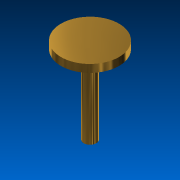
# Autodesk Inventor part: Omron SS-01GL2-E Microswitch Roller Pin
Saved by Autodesk Inventor 2016 (Build 200138000, 138)
## iProperties
Created: 2012-05-23
Material: Brass
Document SubType Name: Modeling
Designer: sdarley
Density: 1 g/cm^3
Project: Microswitch - Omron SS-01GL2-E
Description: Omron SS-01GL2-E Microswitch Roller Pin
Appearance: Brass - Polished
Author: sdarley
Title: Omron SS-01GL2-E Microswitch Roller Pin
Revision Number: 1
Autodesk Inventor part; units mm, degrees
ref_plane "YZ Plane" through (0, 0, 0) normal (1, 0, 0) x (0, 1, 0)
ref_plane "XZ Plane" through (0, 0, 0) normal (0, 1, 0) x (-1, 0, 0)
ref_plane "XY Plane" through (0, 0, 0) normal (0, 0, 1) x (1, 0, 0)
sketch "Sketch1" plane through (0, 0, 0) normal (0, 0, 1) x (1, 0, 0)
  circle A0 centre (0, 0) radius 1.5
  dimension "d0" = 3
  constraints: 1 centre point, 1 coincident
  measures "d0" diameter of A0
extrude "Extrusion1" add sketch "Sketch1" along normal blind 0.4
sketch "Sketch2" plane through (0, 0, 0) normal (0, 0, -1) x (-1, 0, 0)
  circle A0 centre (0, 0) radius 1.5 projected
  circle A1 centre (0, 0) radius 0.5
  dimension "d3" = 1
  constraints: 1 centre point, 1 coincident
  measures "d3" diameter of A1
extrude "Extrusion2" add sketch "Sketch2" along normal blind 4.05 contours A1
sketch "Sketch3" plane through (0, 0, -4.05) normal (0, 0, -1) x (-1, 0, 0)
  circle A0 centre (0, 0) radius 0.5 projected
  circle A1 centre (0, 0) radius 0.85
  dimension "d7" = 1.7
  constraints: 1 centre point, 1 coincident
  measures "d7" diameter of A1
extrude "Extrusion3" add sketch "Sketch3" along normal blind 0.3 contours A0 | A1
sketch "Sketch4" plane through (0, 0, -4.35) normal (0, 0, -1) x (-1, 0, 0)
  circle A0 centre (0, 0) radius 0.85 projected
  circle A1 centre (0, 0) radius 0.45
  dimension "d10" = 0.9
  constraints: 1 centre point, 1 coincident
  measures "d10" diameter of A1
extrude "Extrusion4" cut sketch "Sketch4" against normal blind 0.5 contours A1
body "Solid1"
